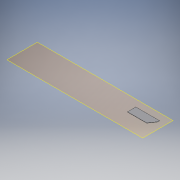
# Autodesk Inventor part: svejselære 2 del 2xxx
Saved by Autodesk Inventor 2018 (Build 220112000, 112)
## iProperties
Created: 2019-10-09
Part Number: svejselære 2 del 2xxx
Material: Generic
Document SubType Name: Sheet Metal
Designer: loppen
Density: 1 g/cm^3
Sheet Metal Rule: Default_mm
Appearance: Default
Author: loppen
Autodesk Inventor part; units mm, degrees
ref_plane "YZ Plane" through (0, 0, 0) normal (1, 0, 0) x (0, 1, 0)
ref_plane "XZ Plane" through (0, 0, 0) normal (0, 1, 0) x (-1, 0, 0)
ref_plane "XY Plane" through (0, 0, 0) normal (0, 0, 1) x (1, 0, 0)
ref_plane "Work Plane1" through (0, 0, 0) normal (0, 0, 1) x (1, 0, 0)
sketch "Sketch1" plane through (0, 0, 0) normal (0, 0, 1) x (1, 0, 0)
  line L0 (820.7818, 193.6487) -> (1020.7818, 193.6487)
  line L1 (1020.7818, 193.6487) -> (1020.7818, 173.6487)
  line L2 (1020.7818, 173.6487) -> (880.2582, -32.3513)
  line L3 (880.2582, -32.3513) -> (820.7818, -32.3513)
  line L4 (820.7818, -32.3513) -> (820.7818, 193.6487)
  point P0 (0, 0)
  dimension "d0" = 55.7
  dimension "d2" = 200
  dimension "d3" = 20
  dimension "d4" = 226
  measures "d0" angle of L0 L2
  measures "d2" distance of L0.start L0.end
  measures "d3" distance of L0.end L1.end
  measures "d4" distance of L3.end L0.start
extrude "Plate1" add sketch "Sketch1" along normal blind 2
equation "\"d1\" = Thickness"
equation "\"BendRadius\" = Thickness"
equation "\"BendReliefWidth\" = Thickness"
equation "\"BendReliefDepth\" = 0.5 * Thickness"
equation "\"CornerReliefSize\" = 4 * Thickness"
equation "\"MinimumRemnant\" = 2 * Thickness"
equation "\"TransitionRadius\" = BendRadius"
equation "\"JacobiRadiusSize\" = BendRadius"
equation "\"GapSize\" = Thickness"
equation "\"Thickness\" = 2"
body "Solid1"
